middleproximalphalanx (Autodesk Fusion 360 design; units mm, degrees)
Autodesk Fusion 360 part; units mm, degrees
sketch "Sketch1" plane through (0, 0, 0) normal (0, 0, 1) x (1, 0, 0)
  line L0 (17.5, 5) -> (-17.5, 5)
  line L1 (-17.5, 5) -> (-17.5, -5)
  line L2 (-17.5, -5) -> (17.5, -5)
  line L3 (17.5, -5) -> (17.5, 5)
  line L4 (17.5, 5) -> (-17.5, -5) construction
  line L5 (-17.5, 5) -> (17.5, -5) construction
  circle A0 centre (17.5, 0) radius 5
  circle A1 centre (-25, 0) radius 10
  circle A2 centre (19.1583, 2.5) radius 0.75
  line L6 (-17.5, 5) -> (17.5, 5)
  line L7 (17.5, 5) -> (17.5, 6)
  line L8 (17.5, 6) -> (-17.5, 6)
  line L9 (-17.5, 6) -> (-17.5, 5)
  circle A3 centre (-25, 0) radius 5
  line L10 (12.5, 0) -> (12.5, 5)
  line L11 (12.5, 0) -> (12.5, -5)
  circle A4 centre (17.5, 0) radius 0.85
  line L12 (-12, -1.75) -> (8, -1.75)
  arc A5 (8, -1.75) -> (8, 1.75) centre (8, 0) ccw
  line L13 (8, 1.75) -> (-12, 1.75)
  arc A6 (-12, 1.75) -> (-12, -1.75) centre (-12, 0) ccw
  line L14 (-12, 0) -> (8, 0) construction
  circle A7 centre (19.1583, 2.5) radius 1.5
  spline S0 degree 5 poles (18.7679, 4.8366) (18.6458, 4.7875) (18.4114, 4.6871) (18.0898, 4.529) (17.7213, 4.3036) (17.3609, 3.9967) (17.0985, 3.6633) (16.927, 3.3012) (16.8328, 2.9069) (16.7939, 2.476) (16.7846, 2.0048) (16.7788, 1.4917) (16.7535, 0.939) (16.6931, 0.3548) (16.5898, -0.247) (16.4416, -0.8499) (16.2502, -1.436) (16.0196, -1.9886) (15.7543, -2.4939) (15.4574, -2.9437) (15.1314, -3.3337) (14.8483, -3.5968) (14.6238, -3.7665) (14.4687, -3.8675) (14.3898, -3.9149) knots 0 0 0 0 0 0 0.05 0.1 0.15 0.2 0.25 0.3 0.35 0.4 0.45 0.5 0.55 0.6 0.65 0.7 0.75 0.8 0.85 0.9 0.95 1 1 1 1 1 1
  line L15 (14.3898, -3.9149) -> (14.3898, -5)
  circle A8 centre (-25, 0) radius 10.5
  point P0 (16.9738, 3.3661)
  point P1 (16.7638, 1.2313)
  point P2 (16, -2)
  dimension "d1" = 35
  dimension "d2" = 10
  dimension "d6" = 20
  dimension "d7" = 7.5
  dimension "d8" = 5
  dimension "d9" = 1.5
  dimension "d10" = 3
  dimension "d12" = 2.5
  dimension "d13" = 35
  dimension "d14" = 1
  dimension "d15" = 10
  dimension "d31" = 1.7
  dimension "d35" = 3.5
  dimension "d36" = 3.25
  dimension "d37" = 12
  dimension "d38" = 8
  dimension "d47" = 3
  dimension "d57" = 21
  constraint horizontal L0
  constraint perpendicular L0 L1
  constraint parallel L0 L2
  constraint parallel L1 L3
  constraint coincident L4 origin
  constraint coincident L5 origin
  constraint midpoint L3 A0.centre
  constraint coincident L2.end A0
  constraint horizontal L6
  constraint vertical L7
  constraint horizontal L8
  constraint vertical L9
  constraint concentric A1 A3
  constraint coincident A0 L10.start
  constraint coincident L0 L10.end
  constraint tangent A0 L10
  constraint perpendicular L0 L10
  constraint coincident L2 L11.end
  constraint tangent A0 L11
  constraint concentric A0 A4
  constraint tangent L12 A5
  constraint tangent A5 L13
  constraint parallel L12 L13
  constraint tangent L13 A6
  constraint tangent L12 A6
  constraint perpendicular L10 L14
  constraint concentric A2 A7
  constraint coincident A0 S0.start
  constraint coincident A0 S0.end
  constraint coincident L2 L15.end
  constraint perpendicular L2 L15
  constraint concentric A1 A8
  measures "d1" distance of L1.end L2.end
  measures "d2" distance of L0.end L1.end
  measures "d6" diameter of A1
  measures "d7" distance of L1 A1.centre
  measures "d8" distance of L2 A1.centre
  measures "d9" diameter of A2
  measures "d10" distance of A0.centre A2.centre
  measures "d12" vertical distance of A0.centre A2.centre
  measures "d13" distance of L0.end L0.start
  measures "d14" distance of L0.end L8.end
  measures "d15" diameter of A3
  measures "d31" diameter of A4
  measures "d35" diameter of A5
  measures "d36" distance of L0 L13
  measures "d37" distance of origin A6.centre
  measures "d38" distance of origin A5.centre
  measures "d47" diameter of A7
  measures "d57" diameter of A8
extrude "Extrude1" add sketch "Sketch1" along normal blind 3 contours L0 A0 L6 L10 | L3 A0 S0 | L3 A0 S0 | L0 L6 L7 L8 A8 | L0 L2 L6 L10 L11 A8 | L3 A0 A4 S0 | L3 A0 A4 S0 | L2 A0 L11 L15 | L0 L2 A1 L6 A8 | L0 A1 L6 L8 A8 | L3 A4 | L3 A4 | L2 A0 L15 | L0 L1 L2 A1 L6 | L0 A1 L6 L8 L9 | L1 L2 A1 L8 L9 | A2 | L12 A5 L13 A6 | A7
extrude "Extrude2" cut sketch "Sketch1" along normal blind 1.5 contours L3 A0 S0 | L3 A0 S0 | L3 A0 A4 S0 | L3 A0 A4 S0 | L3 A4 | L3 A4 | A7
extrude "Extrude3" cut sketch "Sketch1" along normal blind 1.5 contours L2 A0 L11 L15 | L2 A0 L15
extrude "Extrude4" cut sketch "Sketch1" along normal blind 1.5 contours A2
extrude "Extrude5" add sketch "Sketch1" along normal blind 7 contours A2
extrude "Extrude6" cut sketch "Sketch1" along normal blind 1.5 contours A2
extrude "Extrude7" add sketch "Sketch1" along normal blind 1.5 contours L3 A4 | L3 A4
ref_plane "WorkPlane1" through (-6.4638, 0.2545, 5) normal (0, 0, 1) x (1, 0, 0)
mirror "Mirror1" about plane through (-6.4638, 0.2545, 5) normal (0, 0, 1) of bodies 1 merged
extrude "Extrude8" add sketch "Sketch1" along normal blind 7 contours L0 A0 L6 L10 | L0 L6 L7 L8 A8 | L0 L2 L6 L10 L11 A8 | L0 L2 A1 L6 A8 | L0 A1 L6 L8 A8
extrude "Extrude9" cut sketch "Sketch1" along normal blind 15 contours L12 A5 L13 A6
fillet "Fillet2" radius 10 4 edges at (-16.3397, -5, 8.5) (-16.3397, -5, 1.5) (-17, 6, 8.5) (-17, 6, 1.5)
extrude "Extrude10" add sketch "Sketch1" along normal blind 4 from surface at 3 contours L3 A0 S0 | L3 A0 S0 | L2 A0 L11 L15
fillet "Fillet3" radius 10 1 edges at (14.3898, -3.9149, 5)
fillet "Fillet5" radius 8 2 edges at (12.5, -5, 9.25) (12.5, -5, 0.75)
extrude "Extrude11" cut sketch "Sketch1" along normal blind 7 contours L0 L2 A1 L6 A8
extrude "Extrude12" add sketch "Sketch1" along normal blind 3 contours L0 L2 A1 L6 A8
extrude "Extrude13" cut sketch "Sketch1" along normal blind 7 contours L0 A1 L6 L8 L9
extrude "Extrude14" cut sketch "Sketch1" along normal blind 7 contours L0 A1 L6 L8 A8
extrude "Extrude15" add sketch "Sketch1" along normal blind 3 contours L0 A1 L6 L8 A8 | L0 A1 L6 L8 L9
fillet "Fillet8" radius 1 2 faces at (4.1667, 4.5833, 0) (4.1667, 4.5833, 10)
move_face "OffsetFaces1" [suppressed]
move_face "OffsetFaces2" [suppressed]
move_face "OffsetFaces3" [suppressed]
move_face "OffsetFaces4" [suppressed]
move_face "OffsetFaces5" [suppressed]
move_face "OffsetFaces6" [suppressed]
move_face "OffsetFaces7" [suppressed]
delete_face "DeleteFace1" [suppressed]
fillet "Fillet6" [suppressed]
fillet "Fillet7" [suppressed]
equation "d1 = length"
equation "d2 = thickness"
equation "length = 35 mm"
equation "thickness = 10 mm"
equation "gap = 0.3 mm"
equation "d13 = length"
equation "d31 = 2 mm - gap"
equation "d69 = -gap"
equation "d70 = -gap"
equation "d71 = -gap"
equation "d72 = -gap"
equation "d73 = -gap"
equation "d74 = -gap"
